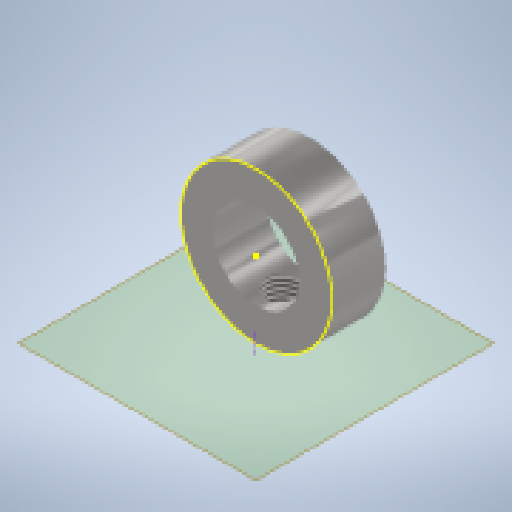
# Autodesk Inventor part: セットカラーSSCCJ8-5
Saved by Autodesk Inventor 2024 (Build 280153000, 153)
## iProperties
Created: 2023-06-01
Part Number: セットカラーSSCCJ8-5
Material: ステンレス鋼
Document SubType Name: Modeling
Designer: yuta2
Density: 8 g/cm^3
Appearance: 半つや出し
Author: yuta2
Autodesk Inventor part; units mm, degrees
ref_plane "YZ Plane" through (0, 0, 0) normal (1, 0, 0) x (0, 1, 0)
ref_plane "XZ Plane" through (0, 0, 0) normal (0, 1, 0) x (-1, 0, 0)
ref_plane "XY Plane" through (0, 0, 0) normal (0, 0, 1) x (1, 0, 0)
sketch "スケッチ1" plane through (0, 0, 0) normal (0, 0, 1) x (1, 0, 0)
  circle A0 centre (0, 0) radius 4
  circle A1 centre (0, 0) radius 7
  dimension "d0" = 8
  dimension "d1" = 14
  constraints: 2 centre point, 2 coincident
  measures "d0" diameter of A0
  measures "d1" diameter of A1
extrude "押し出し1" add sketch "スケッチ1" along normal blind 5
sketch "スケッチ2" plane through (0, 0, 5) normal (0, 0, 1) x (1, 0, 0)
  circle A0 centre (0, 0) radius 7 projected
  point P0 (0, -7)
  constraints: 1 vertical alignment, 1 other
ref_plane "作業平面1" through (0, -7, 5) normal (0, -1, 0) x (1, 0, 0)
sketch "スケッチ3" plane through (0, -7, 5) normal (0, -1, 0) x (1, 0, 0)
  line L0 (7, 0) -> (-7, 0) projected
  line L1 (0, 0) -> (0, -5)
  point P0 (0, -2.5)
  constraints: 2 end point, 2 midpoint, 1 vertical
hole "穴1" at (0, -7, 2.5) direction (0, 1, 0) diameter 3 depth 8 tip angle 118
thread "ねじ1" size "M3x0.5" class "6H" standard "ANSI Metric M Profile" full length
